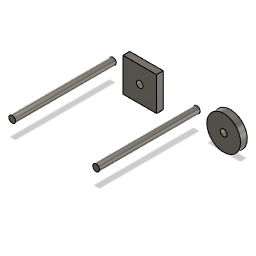
4. ジョイント 回転・スライダ (Autodesk Fusion 360 design; units mm, degrees)
Autodesk Fusion 360 part; units mm, degrees
sketch "スケッチ1" plane through (0, 0, 0) normal (0, 0, 1) x (1, 0, 0)
  circle A0 centre (0, 0) radius 1
  circle A1 centre (35, 0) radius 5
  circle A2 centre (35, 0) radius 1
  line L0 (15, 5) -> (5, 5)
  line L1 (5, 5) -> (5, -5)
  line L2 (5, -5) -> (15, -5)
  line L3 (15, -5) -> (15, 5)
  line L4 (15, 5) -> (5, -5) construction
  line L5 (5, 5) -> (15, -5) construction
  circle A3 centre (10, 0) radius 1
  point P0 (10, 0)
  constraint coincident A0.centre origin
  constraint concentric A1 A2
  constraint horizontal L0
  constraint perpendicular L0 L1
  constraint parallel L0 L2
  constraint parallel L1 L3
  constraint coincident L4 P0
  constraint coincident L5 P0
  constraint coincident P0 A3.centre
extrude "押し出し1" add sketch "スケッチ1" along normal blind 2 contours A1 makes body 1 in component "円盤"
extrude "押し出し1'" add sketch "スケッチ1" along normal blind 30 separate body contours A0 makes body 2 in component "軸"
extrude "押し出し1''" add sketch "スケッチ1" along normal blind 2 separate body contours L0 L1 L2 L3 makes body 3 in component "四角"
component "円盤" placed x (1, 0, 0) y (0, 1, 0) z (0, 0, 1) at (0, 0, 0)
component "軸" placed x (1, 0, 0) y (0, 1, 0) z (0, 0, 1) at (0, 0, 0)
component "四角" placed x (1, 0, 0) y (0, 1, 0) z (0, 0, 1) at (0, 0, 0)
component "軸" placed x (1, 0, 0) y (0, 1, 0) z (0, 0, 1) at (25, 0, 0)
